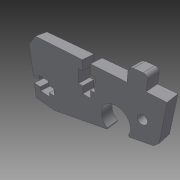
# Autodesk Inventor part: x_carryage_brace_bottom
Saved by Autodesk Inventor 2014 (Build 180170000, 170)
## iProperties
Created: 2014-03-27
Part Number: x_carryage_brace_bottom
Material: Plywood, Finish
Document SubType Name: Modeling
Designer: buben
Density: 0.552 g/cm^3
Appearance: Plywood - New
Author: buben
Autodesk Inventor part; units mm, degrees
ref_plane "YZ Plane" through (0, 0, 0) normal (1, 0, 0) x (0, 1, 0)
ref_plane "XZ Plane" through (0, 0, 0) normal (0, 1, 0) x (-1, 0, 0)
ref_plane "XY Plane" through (0, 0, 0) normal (0, 0, 1) x (1, 0, 0)
sketch "Sketch1" plane through (0, 0, 0) normal (0, 1, 0) x (-1, 0, 0)
  line L0 (0, -37.5) -> (0, 0)
  line L1 (0, 0) -> (-74.5, 0)
  line L2 (-74.5, 0) -> (-74.5, -20)
  line L3 (-74.5, -20) -> (-15, -37.5)
  line L4 (-15, -37.5) -> (0, -37.5)
  dimension "d0" = 37.5
  dimension "d1" = 74.5
  dimension "d2" = 20
  dimension "d3" = 15
  constraints: 10 end point, 2 parallel, 1 perpendicular, 1 vertical
  measures "d0" distance of L0.start L0.end
  measures "d1" distance of L0.end L1.end
  measures "d2" distance of L1.end L2.end
  measures "d3" distance of L3.end L0.start
extrude "Extrusion1" add sketch "Sketch1" along normal blind 6.5
sketch "Sketch2" plane through (0, 0, 0) normal (0, -1, 0) x (1, 0, 0)
  line L0 (0, 0) -> (0, -37.5) projected
  line L1 (0, -37.5) -> (15, -37.5) projected
  line L2 (16.3, -23.5) -> (16.3, -28)
  line L3 (0, -28) -> (0, -23.5)
  line L4 (5, -21) -> (12.3, -21)
  line L5 (12.3, -30.5) -> (5, -30.5)
  line L6 (0, -23.5) -> (5, -23.5)
  line L7 (12.3, -23.5) -> (16.3, -23.5)
  line L8 (16.3, -28) -> (12.3, -28)
  line L9 (5, -28) -> (0, -28)
  line L10 (5, -30.5) -> (5, -28)
  line L11 (5, -23.5) -> (5, -21)
  line L12 (12.3, -21) -> (12.3, -23.5)
  line L13 (12.3, -28) -> (12.3, -30.5)
  point P0 (16.3, -25.75)
  dimension "d6" = 4.5
  dimension "d7" = 2.5
  dimension "d8" = 5
  dimension "d9" = 7.3
  dimension "d10" = 4
  dimension "d12" = 14
  constraints: 24 end point, 10 parallel, 6 collinear, 4 perpendicular, 3 horizontal, 1 midpoint
  measures "d6" distance of L2.start L2.end
  measures "d7" distance of L8.end L5.start
  measures "d8" distance of L9.start L3.start
  measures "d9" distance of L5.start L5.end
  measures "d10" distance of L2.end L8.end
  measures "d12" distance between parallel lines of L6 L1
extrude "Extrusion2" cut sketch "Sketch2" against normal through all
sketch "Sketch3" plane through (0, 0, 0) normal (0, -1, 0) x (1, 0, 0)
  line L0 (74.5, -20) -> (74.5, 0) projected
  line L1 (74.5, 0) -> (0, 0) projected
  line L2 (66.5, 0) -> (58.5, 0)
  line L3 (58.5, 0) -> (58.5, 4.5)
  line L4 (60.5, 6.5) -> (64.5, 6.5)
  line L5 (66.5, 4.5) -> (66.5, 0)
  arc A0 (60.5, 6.5) -> (58.5, 4.5) centre (60.5, 4.5) ccw
  arc A1 (66.5, 4.5) -> (64.5, 6.5) centre (64.5, 4.5) ccw
  dimension "d15" = 2
  dimension "d16" = 8
  dimension "d17" = 6.5
  dimension "d18" = 8
  constraints: 8 end point, 4 point on circle, 4 tangent, 2 centre point, 2 parallel, 1 equal radius, 1 horizontal, 1 perpendicular, 1 point on line
  measures "d15" radius of A0
  measures "d16" distance between parallel lines of L5 L3
  measures "d17" distance between parallel lines of L1 L4
  measures "d18" distance between parallel lines of L0 L5
extrude "Extrusion3" add sketch "Sketch3" against normal blind 6.5
sketch "Sketch4" plane through (0, 0, 0) normal (0, -1, 0) x (1, 0, 0)
  line L0 (58.5, 4.5) -> (58.5, 0) projected
  line L1 (58.5, 0) -> (0, 0) projected
  line L2 (36.25, 0) -> (40.75, 0)
  line L3 (40.75, -16.3) -> (36.25, -16.3)
  line L4 (43.25, -5) -> (43.25, -12.3)
  line L5 (33.75, -12.3) -> (33.75, -5)
  line L6 (33.75, -5) -> (36.25, -5)
  line L7 (40.75, -5) -> (43.25, -5)
  line L8 (43.25, -12.3) -> (40.75, -12.3)
  line L9 (36.25, -12.3) -> (33.75, -12.3)
  line L10 (36.25, -16.3) -> (36.25, -12.3)
  line L11 (36.25, -5) -> (36.25, 0)
  line L12 (40.75, 0) -> (40.75, -5)
  line L13 (40.75, -12.3) -> (40.75, -16.3)
  point P0 (38.5, -16.3)
  dimension "d21" = 4.5
  dimension "d22" = 2.5
  dimension "d23" = 5
  dimension "d24" = 4
  dimension "d25" = 7.3
  dimension "d26" = 20
  constraints: 24 end point, 10 parallel, 6 collinear, 4 perpendicular, 3 horizontal, 1 midpoint
  measures "d21" distance of L3.start L3.end
  measures "d22" distance of L9.start L5.start
  measures "d23" distance of L6.end L2.start
  measures "d24" distance of L3.end L9.start
  measures "d25" distance of L5.start L5.end
  measures "d26" distance from line of L0 point (38.5, -16.3)
extrude "Extrusion4" cut sketch "Sketch4" against normal through all
sketch "Sketch6" plane through (0, 6.5, 0) normal (0, 1, 0) x (1, 0, 0)
  line L0 (40.75, 0) -> (58.5, 0) projected
  line L1 (74.5, 0) -> (74.5, 20) projected
  line L2 (74.5, 20) -> (15, 37.5) projected
  arc A0 (51.3532, 26.8079) -> (60.8316, 24.0201) centre (54.5, 20) ccw
  circle A1 centre (54.5, 20) radius 4 construction
  line L3 (51.3532, 26.8079) -> (60.8316, 24.0201)
  dimension "d34" = 15
  dimension "d35" = 8
  dimension "d36" = 20
  dimension "d37" = 20
  constraints: 2 centre point, 2 end point, 2 point on circle, 2 point on line, 1 coincident, 1 collinear
  measures "d34" diameter of A0
  measures "d35" diameter of A1
  measures "d36" distance from line of A1.centre L1
  measures "d37" distance from line of L0 A0.centre
extrude "Extrusion6" cut sketch "Sketch6" against normal through all
chamfer "Chamfer1" distance 1 angle 45 2 edges at (51.3532, 3.25, -26.8079) (60.8316, 3.25, -24.0201)
chamfer "Chamfer2" distance 2 angle 45 1 edges at (74.5, 3.25, -20)
chamfer "Chamfer3" distance 6 angle 45 1 edges at (0, 3.25, 0)
sketch "Sketch7" plane through (0, 6.5, 0) normal (0, 1, 0) x (1, 0, 0)
  line L0 (66.5, 0) -> (74.5, 0) projected
  line L1 (74.5, 0) -> (74.5, 18) projected
  circle A0 centre (66.5, 12) radius 2.25
  point P0 (0, 0)
  dimension "d49" = 4.5
  dimension "d50" = 8
  dimension "d51" = 12
  constraints: 1 centre point
  measures "d49" diameter of A0
  measures "d50" distance from line of L1 A0.centre
  measures "d51" distance from line of L0 A0.centre
extrude "Extrusion7" cut sketch "Sketch7" against normal through all
body "Solid1"
